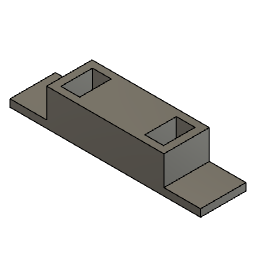
power_board_solder_template v3 (Autodesk Fusion 360 design; units mm, degrees)
Autodesk Fusion 360 part; units mm, degrees
sketch "Sketch1" plane through (0, 0, 0) normal (0, 1, 0) x (1, 0, 0)
  line L0 (16, -6.2) -> (-16, -6.2)
  line L1 (-16, -6.2) -> (-16, 6.2)
  line L2 (-16, 6.2) -> (16, 6.2)
  line L3 (16, 6.2) -> (16, -6.2)
  line L4 (16, -6.2) -> (-16, 6.2) construction
  line L5 (-16, -6.2) -> (16, 6.2) construction
  line L6 (14, 6.2) -> (14, -6.2)
  line L7 (-14, 6.2) -> (-14, -6.2)
  line L8 (8.9, 6.2) -> (8.9, -6.2)
  line L9 (-8.9, 6.2) -> (-8.9, -6.2)
  line L10 (-16, 6.2) -> (-26, 6.2)
  line L11 (-26, 6.2) -> (-26, -6.2)
  line L12 (-26, -6.2) -> (-16, -6.2)
  line L13 (-16, -6.2) -> (-16, 6.2)
  line L14 (16, 6.2) -> (26, 6.2)
  line L15 (26, 6.2) -> (26, -6.2)
  line L16 (26, -6.2) -> (16, -6.2)
  line L17 (16, -6.2) -> (16, 6.2)
  line L18 (-26, 4.3) -> (26, 4.3)
  line L19 (-26, -4.3) -> (26, -4.3)
  dimension "d1" = 32
  dimension "d2" = 12.4
  dimension "d3" = 2
  dimension "d4" = 2
  dimension "d5" = 5.1
  dimension "d6" = 5.1
  dimension "d7" = 10
  dimension "d8" = 10
  dimension "d13" = 1.9
  dimension "d14" = 1.9
  constraint horizontal L0
  constraint perpendicular L0 L1
  constraint parallel L0 L2
  constraint parallel L1 L3
  constraint coincident L4 origin
  constraint coincident L5 origin
  constraint coincident L2 L6.start
  constraint coincident L0 L6.end
  constraint perpendicular L0 L6
  constraint coincident L2 L7.start
  constraint coincident L0 L7.end
  constraint perpendicular L0 L7
  constraint coincident L2 L8.start
  constraint coincident L0 L8.end
  constraint perpendicular L0 L8
  constraint coincident L2 L9.start
  constraint coincident L0 L9.end
  constraint perpendicular L0 L9
  constraint horizontal L10
  constraint vertical L11
  constraint horizontal L12
  constraint vertical L13
  constraint horizontal L14
  constraint vertical L15
  constraint horizontal L16
  constraint vertical L17
  constraint coincident L0.end L12
  constraint coincident L0.start L16
  constraint coincident L11 L18.start
  constraint coincident L15 L18.end
  constraint perpendicular L15 L18
  constraint coincident L11 L19.start
  constraint coincident L15 L19.end
  constraint perpendicular L15 L19
  measures "d1" distance of L1.end L2.end
  measures "d2" distance of L0.end L1.end
  measures "d3" distance of L3 L6
  measures "d4" distance of L1 L7
  measures "d5" distance of L6 L8
  measures "d6" distance of L7 L9
  measures "d7" distance of L15 L17
  measures "d8" distance of L11 L13
  measures "d13" distance of L2 L18
  measures "d14" distance of L0 L19
extrude "Extrude1" add sketch "Sketch1" along normal blind 2
extrude "Extrude2" add sketch "Sketch1" along normal blind 10 contours L0 L3 L6 L17 L19 | L3 L6 L17 L18 L19 | L0 L8 L9 L19 | L2 L3 L6 L17 L18 | L8 L9 L18 L19 | L0 L1 L7 L13 L19 | L2 L8 L9 L18 | L1 L7 L13 L18 L19 | L1 L2 L7 L13 L18
extrude "Extrude3" add sketch "Sketch1" along normal up to surface (10 mm away) contours L0 L6 L8 L19 | L0 L7 L9 L19 | L2 L6 L8 L18 | L2 L7 L9 L18
